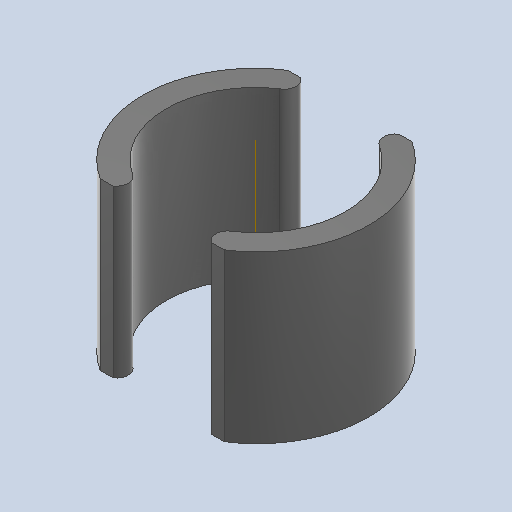
# Autodesk Inventor part: Imãs
Saved by Autodesk Inventor 2022.2 (Build 262287000, 287)
## iProperties
Created: 2021-01-23
Part Number: Imãs
Material: Genérico
Document SubType Name: Modeling
Designer: João
Density: 1 g/cm^3
Appearance: Padrão
Mass: 0.225857 g
Surface Area: 4.62783 cm^2
Volume: 0.225857 cm^3
Author: João
Autodesk Inventor part; units mm, degrees
ref_plane "YZ Plane" through (0, 0, 0) normal (1, 0, 0) x (0, 1, 0)
ref_plane "XZ Plane" through (0, 0, 0) normal (0, 1, 0) x (-1, 0, 0)
ref_plane "XY Plane" through (0, 0, 0) normal (0, 0, 1) x (1, 0, 0)
sketch "Esboço1" plane through (0, 0, 0) normal (0, 1, 0) x (-1, 0, 0)
  line L0 (3.2233, 5.0079) -> (-3.2768, 5.0079)
  line L1 (-3.2767, -4.9922) -> (3.2232, -4.9922)
  arc A0 (3.2232, -4.9922) -> (3.2233, 5.0079) centre (0.0528, 0.0079) ccw
  arc A1 (-3.2768, 5.0079) -> (-3.2767, -4.9922) centre (-0.1063, 0.0079) ccw
  line L2 (3.2233, 5.0079) -> (-3.2768, 5.0079)
  line L3 (-3.2767, -4.9922) -> (3.2232, -4.9922)
  line L4 (3.1646, -4.7922) -> (-3.2181, -4.7922)
  arc A2 (-3.2182, 4.8079) -> (-3.2181, -4.7922) centre (-0.1063, 0.0079) ccw
  line L5 (-3.2182, 4.8079) -> (3.1647, 4.8079)
  arc A3 (3.1646, -4.7922) -> (3.1647, 4.8079) centre (0.0528, 0.0079) ccw
  arc A4 (-2.2768, 4.658) -> (-2.0269, 4.808) centre (-2.2768, 4.9413) ccw
  arc A5 (-2.5268, 4.808) -> (-2.2768, 4.658) centre (-2.2768, 4.9413) ccw
  line L6 (-0.0267, 5.0079) -> (-0.0267, 0.0079)
  line L7 (-0.0267, 5.0079) -> (4.9733, 5.0079) construction
  line L8 (-0.0267, 0.0079) -> (-0.0267, -4.9922)
  line L9 (-0.0267, 0.0079) -> (-6.0268, 0.0078)
  line L10 (-0.0267, 0.0079) -> (5.9733, 0.0078)
  arc A6 (-2.0267, -4.7922) -> (-2.2767, -4.6422) centre (-2.2767, -4.9255) ccw
  arc A7 (-2.2767, -4.6422) -> (-2.5267, -4.7922) centre (-2.2767, -4.9255) ccw
  line L11 (-0.0266, -4.9921) -> (-0.0267, 0.0079)
  arc A8 (2.2232, -4.6422) -> (1.9732, -4.7922) centre (2.2232, -4.9255) ccw
  arc A9 (2.4732, -4.7922) -> (2.2232, -4.6422) centre (2.2232, -4.9255) ccw
  arc A10 (1.9734, 4.808) -> (2.2234, 4.658) centre (2.2233, 4.9413) ccw
  arc A11 (2.2234, 4.658) -> (2.4733, 4.808) centre (2.2233, 4.9413) ccw
  arc A12 (2.5118, -3.7852) -> (2.5119, 3.801) centre (0.0528, 0.0079) ccw
  arc A13 (2.5501, -3.7602) -> (2.5082, -4.7922) centre (2.8382, -4.2887) ccw
  arc A14 (2.5083, 4.8079) -> (2.5502, 3.7759) centre (2.8383, 4.3045) ccw
  dimension "d21" = 0.2
  dimension "d22" = 0.2
  dimension "d23" = 0.2
  dimension "d24" = 0.2
  dimension "d28" = 1
  dimension "d29" = 5
  dimension "d30" = 90
  dimension "d31" = 1
  dimension "d32" = 1
  dimension "d33" = 1
  constraints: 34 point on circle, 24 end point, 16 symmetric about line, 15 centre point, 3 horizontal, 2 midpoint, 2 parallel, 2 point on line, 2 tangent, 1 perpendicular, 1 vertical, 6 other
  measures "d21" distance between parallel lines of L1 L4
  measures "d22" distance between parallel lines of L0 L5
  measures "d23" radial gap between concentric circles of A3 A0
  measures "d24" radial gap between concentric circles of A1 A2
  measures "d28" horizontal distance of L2.end A4.centre
  measures "d29" distance of L6.start L6.end
  measures "d30" angle of L6 L7
  measures "d31" horizontal distance of L2.start A11.centre
  measures "d32" horizontal distance of L3.end A9.centre
  measures "d33" horizontal distance of L3.start A6.centre
extrude "Extrusão1" add sketch "Esboço1" along normal blind 8.5 contours L10 A12 A14 L5 A3 | A3 L4 A13 A12 L10
pattern_circular "Padrão circular1" count 2 over 360 about axis through (0, -10, 0) along (0, 1, 0) of "Extrusão1"
